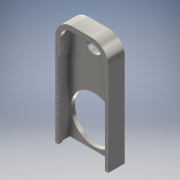
# Autodesk Inventor part: Cup_Dispenser_Hull
Saved by Autodesk Inventor 2016 (Build 200138000, 138)
## iProperties
Created: 2015-07-04
Part Number: Cup_Dispenser_Hull
Material: Generic
Document SubType Name: Modeling
Designer: marku
Density: 1 g/cm^3
Appearance: Titanium
Author: marku
Autodesk Inventor part; units mm, degrees
ref_plane "YZ Plane" through (0, 0, 0) normal (1, 0, 0) x (0, 1, 0)
ref_plane "XZ Plane" through (0, 0, 0) normal (0, 1, 0) x (-1, 0, 0)
ref_plane "XY Plane" through (0, 0, 0) normal (0, 0, 1) x (1, 0, 0)
derived "Cup_Dispenser_Slider.ipt"
sketch "Sketch13" plane through (0, 0, 0) normal (0, 1, 0) x (-1, 0, 0)
  circle A0 centre (0, 0) radius 35 construction
  circle A1 centre (0, 0) radius 31.375 construction
  line L0 (0, 60.7625) -> (0, -56.1294) construction
  line L1 (45.182, 0) -> (-48.0239, 0) construction
  circle A2 centre (0, 35) radius 35 construction
  circle A3 centre (0, 35) radius 31.375 construction
  line L2 (31.375, 35) -> (31.375, 19.4884)
  line L3 (35, 19.4884) -> (35, 70)
  line L4 (35, 70) -> (0, 70)
  line L5 (31.375, 19.4884) -> (35, 19.4884)
  arc A4 (31.375, 35) -> (0, 66.375) centre (0, 35) ccw
  line L6 (0, 70) -> (0, 66.375) construction
  line L7 (0, 31.375) -> (0, 3.625) construction
  line L8 (0, 17.5) -> (45.182, 17.5) construction
  line L9 (-35, 19.4884) -> (-35, 70)
  line L10 (-35, 70) -> (0, 70)
  line L11 (-31.375, 19.4884) -> (-35, 19.4884)
  line L12 (-31.375, 35) -> (-31.375, 19.4884)
  arc A5 (0, 66.375) -> (-31.375, 35) centre (0, 35) ccw
  line L13 (35, 15.5116) -> (35, -35)
  line L14 (31.375, 15.5116) -> (35, 15.5116)
  line L15 (31.375, 0) -> (31.375, 15.5116)
  arc A6 (0, -31.375) -> (31.375, 0) centre (0, 0) ccw
  line L16 (35, -35) -> (0, -35)
  line L17 (-35, -35) -> (0, -35)
  arc A7 (-31.375, 0) -> (0, -31.375) centre (0, 0) ccw
  line L18 (-35, 15.5116) -> (-35, -35)
  line L19 (-31.375, 15.5116) -> (-35, 15.5116)
  line L20 (-31.375, 0) -> (-31.375, 15.5116)
  line L21 (35, 70) -> (35, -35)
  line L22 (-35, -35) -> (-35, 70)
  line L23 (-38, 73) -> (38, 73)
  line L24 (38, 73) -> (38, -38)
  line L25 (38, -38) -> (-38, -38)
  line L26 (-38, -38) -> (-38, 73)
  line L27 (-38, 73) -> (38, -38) construction
  line L28 (38, 73) -> (-38, -38) construction
sketch "Sketch2" plane through (0, 0, 0) normal (0, 1, 0) x (-1, 0, 0)
  line L0 (-41, 76) -> (41, 76)
  line L1 (41, 76) -> (41, -41)
  line L2 (41, -41) -> (-41, -41)
  line L3 (-41, -41) -> (-41, 76)
  line L4 (-41, 76) -> (41, -41) construction
  line L5 (41, 76) -> (-41, -41) construction
  line L6 (38, -38) -> (38, 73)
  line L7 (38, 73) -> (-38, 73)
  line L8 (-38, 73) -> (-38, -38)
  line L9 (-38, -38) -> (38, -38)
  line L10 (-35, 35) -> (35, 35) construction
  line L11 (35, 35) -> (35, -35) construction
  line L12 (35, -35) -> (-35, -35) construction
  line L13 (-35, -35) -> (-35, 35) construction
  line L14 (-35, 35) -> (35, -35) construction
  line L15 (35, 35) -> (-35, -35) construction
  circle A0 centre (0, 0) radius 36
  point P0 (0, 17.5)
  dimension "d1" = 82
  dimension "d2" = 117
  dimension "d3" = 3
  dimension "d4" = 70
  dimension "d5" = 70
  dimension "d8" = 72
  constraints: 32 end point, 6 parallel, 5 coincident, 4 midpoint, 3 perpendicular, 2 horizontal, 1 centre point, 3 other
  measures "d1" distance of L1.end L2.end
  measures "d2" distance of L0.end L1.end
  measures "d3" distance between parallel lines of L1 L6
  measures "d4" distance of L11.end L12.end
  measures "d5" distance of L10.end L11.end
  measures "d8" diameter of A0
extrude "Extrusion1" add sketch "Sketch2" against normal blind 6 contours L0 L1 L2 L3 | L9 L8 L7 L6
hole "Hole1" at (0, 0, 17.5) at (-35, 0, 35) at (-35, 0, -35) at (35, 0, -35) at (35, 0, 35) direction (0, -1, 0) diameter 3 depth 4 tip angle 118
extrude "Extrusion2" add sketch "Sketch2" against normal blind 19.5 contours L0 L1 L2 L3
chamfer "Chamfer1" distance 2 angle 45 2 edges at (-38, -12.75, 73) (38, -12.75, 73)
sketch "Sketch4" plane through (41, 0, -41) normal (0, 0, -1) x (-1, 0, 0)
  line L0 (79, -6) -> (3, -6) projected
  line L1 (79, -6) -> (79, -19.5) projected
  line L2 (3, -6) -> (3, -19.5) projected
  line L3 (3, -19.5) -> (79, -19.5) projected
  point P0 (41, 0)
extrude "Extrusion4" cut sketch "Sketch4" against normal blind 3
sketch "Sketch22" plane through (0, -19.5, 0) normal (0, -1, 0) x (1, 0, 0)
  line L0 (-38, -41) -> (-38, 71) construction
  line L1 (-36, 73) -> (-38, 71) construction
  line L2 (-36, 73) -> (36, 73) projected
  line L3 (38, 71) -> (36, 73) construction
  line L4 (38, 71) -> (38, -41) construction
  line L5 (38, -41) -> (41, -41) projected
  line L6 (41, -41) -> (41, 76) projected
  line L7 (41, 76) -> (-41, 76) projected
  line L8 (-41, 76) -> (-41, -41) projected
  line L9 (-41, -41) -> (-38, -41) projected
  line L10 (38, -41) -> (-38, -41) projected
  line L11 (-36, -41) -> (-36, 0)
  circle A0 centre (0, 0) radius 36 construction
  line L12 (-36, 73) -> (36, 73) projected
  line L13 (-36, 0) -> (-36, 73)
  line L14 (36, -41) -> (36, 0)
  line L15 (36, 73) -> (36, 0)
  line L16 (38, -41) -> (38, 71) construction
  constraints: 8 end point, 3 tangent, 2 point on circle, 2 point on line, 1 parallel, 1 perpendicular
extrude "Extrusion13" add sketch "Sketch22" along normal blind 6 contours L13 L11 L10 L9 L8 L7 L6 L5 L14 L15 L2
sketch "Sketch23" plane through (-41, 0, 76) normal (0, 0, 1) x (1, 0, 0)
  line L0 (77, -19.5) -> (77, -6) projected
  line L1 (77, -19.5) -> (77, -25.5) projected
  line L2 (5, -25.5) -> (77, -25.5) projected
  line L3 (5, -19.5) -> (5, -25.5) projected
  line L4 (5, -6) -> (5, -19.5) projected
  line L5 (77, -6) -> (5, -6) projected
  point P0 (41, 0)
extrude "Extrusion14" cut sketch "Sketch23" against normal blind 3
sketch "Sketch24" plane through (0, 0, 0) normal (0, 1, 0) x (1, 0, 0)
  line L0 (-41, -76) -> (-41, -101.3074)
  arc A0 (-41, -101.3074) -> (-14.5074, -127.8) centre (-14.5074, -101.3074) ccw
  line L1 (-14.5074, -127.8) -> (16, -127.8)
  arc A1 (16, -127.8) -> (41, -102.8) centre (16, -102.8) ccw
  line L2 (41, -102.8) -> (41, -76)
  line L3 (-41, -76) -> (41, -76)
  line L4 (-36, -76) -> (36, -76) projected
  line L5 (-14.5074, -122.8) -> (-14.5074, -127.8) construction
  line L6 (16, -122.8) -> (16, -127.8) construction
  circle A2 centre (0, -99.5) radius 11.5 projected
  point P0 (0, 0)
  point P1 (16, -125.3)
  dimension "d152" = 5
  constraints: 12 end point, 4 point on circle, 4 tangent, 3 vertical, 2 centre point, 2 point on line, 1 collinear, 1 horizontal, 1 midpoint, 1 perpendicular
  measures "d152" distance of L5.start L5.end
extrude "Extrusion15" add sketch "Sketch24" against normal up to surface (6 mm away)
sketch "Sketch25" plane through (0, 0, 0) normal (0, 1, 0) x (1, 0, 0)
  line L0 (-15.5, -115) -> (15.5, -115) construction
  line L1 (15.5, -115) -> (15.5, -84) construction
  line L2 (15.5, -84) -> (-15.5, -84) construction
  line L3 (-15.5, -84) -> (-15.5, -115) construction
  line L4 (-15.5, -115) -> (15.5, -84) construction
  line L5 (15.5, -115) -> (-15.5, -84) construction
  line L6 (-30, -74.75) -> (30, -74.75) construction
  line L7 (30, -74.75) -> (30, -44.75) construction
  line L8 (30, -44.75) -> (-30, -44.75) construction
  line L9 (-30, -44.75) -> (-30, -74.75) construction
  line L10 (-30, -74.75) -> (30, -44.75) construction
  line L11 (30, -74.75) -> (-30, -44.75) construction
  line L12 (11.1915, -41) -> (-11.1915, -41) construction
  line L13 (15.0858, -78.5) -> (-15.0858, -78.5) projected
  line L14 (0, -78.5) -> (0, -74.75) construction
  line L15 (0, -41) -> (0, -44.75) construction
  circle A0 centre (0, -99.5) radius 11.5 construction
  point P0 (0, 0)
  point P1 (0, -59.75)
  dimension "d107" = 31
  dimension "d108" = 31
  dimension "d125" = 60
  dimension "d126" = 30
  constraints: 28 end point, 8 coincident, 8 midpoint, 5 equal length, 2 horizontal, 2 perpendicular, 1 collinear, 1 vertical
  measures "d107" distance of L2.end L1.end
  measures "d108" distance of L1.end L0.end
  measures "d125" distance of L8.end L7.end
  measures "d126" distance of L7.end L6.end
hole "Hole6" at (-15.5, 0, 84) at (-15.5, 0, 115) at (15.5, 0, 115) at (15.5, 0, 84) at (-30, 0, 74.75) at (-30, 0, 44.75) at (30, 0, 44.75) at (30, 0, 74.75) at (0, 0, 74.75) at (0, 0, 44.75) direction (0, -1, 0) diameter 3 depth 4 tip angle 118
sketch "Sketch26" plane through (0, -6, 0) normal (0, -1, 0) x (1, 0, 0)
  line L0 (38, 71) -> (36, 73) construction
  line L1 (36, 76) -> (36, 73) construction
  line L2 (41, 76) -> (36, 76) projected
  line L3 (-36, 76) -> (-36, 73) construction
  line L4 (-36, 73) -> (-38, 71) construction
  line L5 (-38, -41) -> (-38, 71) construction
  line L6 (38, -41) -> (-38, -41) construction
  line L7 (38, -41) -> (38, 71) construction
  circle A0 centre (0, 0) radius 36 construction
  line L8 (-36, 76) -> (36, 76) construction
  line L9 (36, 76) -> (36, 103)
  arc A1 (36, 103) -> (16, 123) centre (16, 103) ccw
  line L10 (16, 123) -> (-16, 123)
  arc A2 (-16, 123) -> (-36, 103) centre (-16, 103) ccw
  line L11 (-36, 76) -> (-36, 73) projected
  line L12 (-36, 103) -> (-36, 76)
  line L13 (41, 102.8) -> (41, 76) projected
  arc A3 (41, 102.8) -> (16, 127.8) centre (16, 102.8) ccw projected
  line L14 (-14.5074, 127.8) -> (16, 127.8) projected
  arc A4 (-14.5074, 127.8) -> (-41, 101.3074) centre (-14.5074, 101.3074) ccw projected
  line L15 (-41, 76) -> (-41, 101.3074) projected
  line L16 (-36, 76) -> (-41, 76) projected
  constraints: 6 end point, 4 point on circle, 2 centre point, 2 tangent, 1 collinear, 1 horizontal, 1 vertical
extrude "Extrusion16" add sketch "Sketch26" along normal up to surface (13.5 mm away)
sketch "Sketch28" plane through (-14.5074, -19.5, 127.8) normal (0, -1, 0) x (1, 0, 0)
  arc A0 (47.5074, -24.8) -> (30.5074, -7.8) centre (30.5074, -24.8) ccw
  line L0 (47.5074, -24.8) -> (47.5074, -48.8)
  line L1 (-18.4926, -48.8) -> (-18.4926, -24.8)
  arc A1 (-1.4926, -7.8) -> (-18.4926, -24.8) centre (-1.4926, -24.8) ccw
  line L2 (-1.4926, -7.8) -> (30.5074, -7.8)
  arc A2 (50.5074, -24.8) -> (30.5074, -4.8) centre (30.5074, -24.8) ccw projected
  line L3 (50.5074, -24.8) -> (50.5074, -51.8) projected
  line L4 (55.5074, -51.8) -> (50.5074, -51.8) projected
  line L5 (55.5074, -51.8) -> (55.5074, -25) projected
  arc A3 (55.5074, -25) -> (30.5074, 0) centre (30.5074, -25) ccw projected
  line L6 (30.5074, 0) -> (0, 0) projected
  arc A4 (0, 0) -> (-26.4926, -26.4926) centre (0, -26.4926) ccw projected
  line L7 (-26.4926, -26.4926) -> (-26.4926, -51.8) projected
  line L8 (-21.4926, -51.8) -> (-26.4926, -51.8) projected
  line L9 (-21.4926, -51.8) -> (-21.4926, -24.8) projected
  arc A5 (-1.4926, -4.8) -> (-21.4926, -24.8) centre (-1.4926, -24.8) ccw projected
  line L10 (-1.4926, -4.8) -> (30.5074, -4.8) projected
  line L11 (47.5074, -48.8) -> (50.5074, -51.8)
  line L12 (-18.4926, -48.8) -> (-21.4926, -51.8)
  point P0 (14.5074, -127.8)
  dimension "d158" = 3
  dimension "d161" = 45
  dimension "d162" = 45
  constraints: 10 end point, 4 point on circle, 4 tangent, 2 centre point, 2 vertical, 1 horizontal
  measures "d158" distance between parallel lines of L3 L0
  measures "d161" angle of L9 L12
  measures "d162" angle of L3 L11
extrude "Extrusion17" add sketch "Sketch28" along normal up to surface (6 mm away)
sketch "Sketch29" plane through (0, 0, 0) normal (0, 1, 0) x (1, 0, 0)
  circle A0 centre (-30, -74.75) radius 1.5 construction
  circle A1 centre (-30, -44.75) radius 1.5 construction
  circle A2 centre (0, -44.75) radius 1.5 construction
  circle A3 centre (0, -74.75) radius 1.5 construction
  circle A4 centre (0, -74.75) radius 1.5 construction
  line L0 (-30, -44.75) -> (0, -74.75) construction
  circle A5 centre (-30, -74.75) radius 1.5 construction
  line L1 (0, -74.75) -> (-30, -74.75) construction
  line L2 (-30, -74.75) -> (0, -44.75) construction
  line L3 (0, -44.75) -> (-30, -44.75) construction
  line L4 (-30, -74.75) -> (-30, -44.75) construction
  line L5 (0, -44.75) -> (0, -74.75) construction
  circle A6 centre (-15, -59.75) radius 12
  line L6 (-3, -59.75) -> (0, -59.75) construction
  circle A7 centre (15, -59.75) radius 12
  point P0 (0, 0)
  dimension "d127" = 3
  constraints: 14 end point, 2 horizontal, 2 midpoint, 2 parallel, 2 perpendicular, 1 centre point, 1 horizontal alignment, 1 symmetric about line, 3 other
  measures "d127" distance of L6.start L6.end
extrude "Extrusion18" cut sketch "Sketch29" against normal blind 2
sketch "Sketch30" plane through (0, -25.5, 0) normal (0, -1, 0) x (1, 0, 0)
  line L0 (36, 76) -> (36, -41) projected
  line L1 (36, -41) -> (41, -41) projected
  line L2 (41, -41) -> (41, 102.8) projected
  line L3 (-41, -41) -> (-41, 101.3074) projected
  line L4 (-41, -41) -> (-36, -41) projected
  line L5 (-36, -41) -> (-36, 76) projected
  line L6 (-38.5, -38) -> (-36, -38) construction
  line L7 (-36, -41) -> (-36, 76) projected
  line L8 (-38.5, -38) -> (-41, -38) construction
  line L9 (-41, -41) -> (-41, 101.3074) projected
  line L10 (0, -89.4665) -> (0, 187.6644) construction
  line L11 (-33, 79) -> (-36, 76) projected
  line L12 (-33, 103) -> (-33, 79) projected
  arc A0 (-16, 120) -> (-33, 103) centre (-16, 103) ccw projected
  line L13 (16, 120) -> (-16, 120) projected
  arc A1 (33, 103) -> (16, 120) centre (16, 103) ccw projected
  line L14 (33, 79) -> (33, 103) projected
  line L15 (36, 76) -> (33, 79) projected
  arc A2 (41, 102.8) -> (16, 127.8) centre (16, 102.8) ccw projected
  line L16 (-14.5074, 127.8) -> (16, 127.8) projected
  arc A3 (-14.5074, 127.8) -> (-41, 101.3074) centre (-14.5074, 101.3074) ccw projected
  point P0 (0, 0)
  point P1 (-36, 70)
  point P2 (-38.5, -26)
  point P3 (-38.5, -14)
  point P4 (-38.5, -2)
  point P5 (-38.5, 10)
  point P6 (-38.5, 22)
  point P7 (-38.5, 34)
  point P8 (-38.5, 46)
  point P9 (-38.5, 58)
  point P10 (38.5, -38)
  point P11 (38.5, -26)
  point P12 (38.5, -14)
  point P13 (38.5, -2)
  point P14 (38.5, 10)
  point P15 (38.5, 22)
  point P16 (38.5, 34)
  point P17 (38.5, 46)
  point P18 (38.5, 58)
  point P19 (-41, 76)
  point P20 (-36, 103)
  dimension "d130" = 3
  dimension "d133" = 12
  dimension "d60" = 31
  dimension "d61" = 31
  dimension "d67" = 23
  dimension "d68" = 3
  dimension "d69" = 23
  constraints: 9 symmetric about line, 6 end point, 4 point on line, 2 vertical, 1 collinear, 1 perpendicular, 8 other
  measures "d130" distance from line of L4 L6.start
  measures "d133" distance of L6.start point (-38.5, -26)
hole "Hole7" at (-38.5, -25.5, -38) at (-38.5, -25.5, -26) at (-38.5, -25.5, -14) at (-38.5, -25.5, -2) at (-38.5, -25.5, 10) at (-38.5, -25.5, 22) at (-38.5, -25.5, 34) at (-38.5, -25.5, 46) at (-38.5, -25.5, 58) at (38.5, -25.5, -38) at (38.5, -25.5, -26) at (38.5, -25.5, -14) at (38.5, -25.5, -2) at (38.5, -25.5, 10) at (38.5, -25.5, 22) at (38.5, -25.5, 34) at (38.5, -25.5, 46) at (38.5, -25.5, 58) direction (0, 1, 0) diameter 2 depth 4 tip angle 118
sketch "Sketch16" plane through (0, 0, 0) normal (0, 1, 0) x (1, 0, 0)
  line L0 (-36, -73) -> (-36, -103) projected
  arc A0 (-36, -103) -> (-16, -123) centre (-16, -103) ccw projected
  line L1 (16, -123) -> (-16, -123) projected
  arc A1 (16, -123) -> (36, -103) centre (16, -103) ccw projected
  line L2 (36, -103) -> (36, -73) projected
  arc A2 (-41, -103) -> (-18, -126) centre (-18, -103) ccw projected
  line L3 (-18, -126) -> (18, -126) projected
  arc A3 (18, -126) -> (41, -103) centre (18, -103) ccw projected
  line L4 (-41, -103) -> (-41, -73)
  line L5 (-41, 41) -> (-41, -103) projected
  line L6 (-36, -73) -> (-41, -73)
  line L7 (41, -103) -> (41, -73)
  line L8 (41, 41) -> (41, -103) projected
  line L9 (36, -73) -> (41, -73)
  point P0 (0, 0)
  constraints: 8 end point, 2 perpendicular, 2 point on line
sketch "Sketch18" plane through (0, 0, 0) normal (0, 1, 0) x (1, 0, 0)
  line L0 (35, -72) -> (-35, -72)
  line L1 (-35, -72) -> (-35, -48)
  line L2 (-35, -48) -> (35, -48)
  line L3 (35, -48) -> (35, -72)
  line L4 (35, -72) -> (-35, -48) construction
  line L5 (-35, -72) -> (35, -48) construction
  line L6 (-41, 41) -> (-41, -103) projected
  line L7 (0, -123) -> (0, -57.6471) construction
  point P0 (0, 0)
  point P1 (0, -60)
  point P2 (0, -72)
  point P3 (0, -48)
  dimension "d81" = 6
  dimension "d96" = 24
  dimension "d97" = 48
  constraints: 12 end point, 4 coincident, 4 midpoint, 2 parallel, 1 horizontal, 1 perpendicular, 1 point on line, 1 other
  measures "d81" distance between parallel lines of L6 L1
  measures "d96" distance between parallel lines of L2 L0
  measures "d97" distance from line of point (0, 0) L2
sketch "Sketch21" plane through (0, 0, 0) normal (0, 1, 0) x (1, 0, 0)
  circle A0 centre (0, -72) radius 1.5 projected
  circle A1 centre (35, -48) radius 1.5 projected
  circle A2 centre (-35, -72) radius 1.5 projected
  circle A3 centre (-35, -48) radius 1.5 projected
  circle A4 centre (35, -72) radius 1.5 projected
  circle A5 centre (0, -48) radius 1.5 projected
  circle A6 centre (-15.5, -115) radius 1.5 projected
  circle A7 centre (-15.5, -84) radius 1.5 projected
  circle A8 centre (15.5, -84) radius 1.5 projected
  circle A9 centre (15.5, -115) radius 1.5 projected
  circle A10 centre (0, 0) radius 36 projected
  line L0 (-41, 41) -> (-41, -103) projected
  arc A11 (-41, -103) -> (-18, -126) centre (-18, -103) ccw projected
  line L1 (-18, -126) -> (18, -126) projected
  arc A12 (18, -126) -> (41, -103) centre (18, -103) ccw projected
  line L2 (41, 41) -> (41, -103) projected
  line L3 (-41, 41) -> (41, 41) projected
  circle A13 centre (35, -35) radius 1.5 projected
  circle A14 centre (-35, 35) radius 1.5 projected
  circle A15 centre (-35, -35) radius 1.5 projected
  circle A16 centre (35, 35) radius 1.5 projected
  circle A17 centre (0, -99.5) radius 11.5 projected
  line L4 (0, -136.0201) -> (0, 47.5544) construction
  circle A18 centre (-18, -60.7956) radius 14.3193
  circle A19 centre (-25.2211, -97.6989) radius 9.0279
  circle A20 centre (18, -60.7956) radius 14.3193
  circle A21 centre (25.2211, -97.6989) radius 9.0279
  constraints: 4 centre point, 2 end point, 2 symmetric about line, 1 point on line, 1 vertical, 2 other
body "Solid1"
